Autodesk Fusion 360 part; units mm, degrees
(part 2 of 3)
component "Output_Shaft" placed x (1, 0, 0) y (0, 1, 0) z (0, 0, 1) at (0, 0, 0)
equation "d46 = d45"

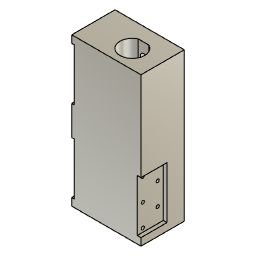
design "主轴连接"
Autodesk Fusion 360 part; units mm, degrees
sketch "草图1" plane through (0, 0, 0) normal (0, 0, 1) x (1, 0, 0)
  line L0 (4.3589, 9) -> (-4.3589, 9)
  arc A0 (-4.3589, 9) -> (4.3589, 9) centre (0, 0) ccw
  line L1 (-34, -15) -> (22, -15)
  line L2 (22, -15) -> (22, 20)
  line L3 (22, 20) -> (-34, 20)
  line L4 (-34, 20) -> (-34, -15)
  line L5 (-34, -15) -> (22, 20) construction
  line L6 (22, -15) -> (-34, 20) construction
  point P0 (-6, 2.5)
  dimension "d1" = 20
  dimension "d2" = 9
  dimension "d3" = 20
  dimension "d29" = 15
  dimension "d30" = 22
  dimension "d31" = 34
  constraint coincident A0.centre origin
  constraint horizontal L0
  constraint horizontal L1
  constraint perpendicular L1 L2
  constraint parallel L1 L3
  constraint parallel L2 L4
  constraint midpoint L5 P0
  measures "d1" diameter of A0
  measures "d2" distance of A0.centre L0
  measures "d3" distance of A0.centre L3
  measures "d29" distance of A0.centre L1
  measures "d30" distance of A0.centre L2
  measures "d31" distance of A0.centre L4
extrude "拉伸1" add sketch "草图1" along normal blind 120
sketch "草图2" plane through (0, 0, 0) normal (0, 1, 0) x (1, 0, 0)
  line L0 (0, 23.9803) -> (0, -42.7721) construction
  circle A0 centre (0, -9.3959) radius 2.5
  circle A1 centre (0, -29.3959) radius 2.5
  circle A2 centre (0, -49.3959) radius 2.5
  circle A3 centre (0, -69.3959) radius 2.5
  circle A4 centre (0, -89.3959) radius 2.5
  circle A5 centre (0, -109.3959) radius 2.5
  dimension "d7" = 5
  dimension "d10" = 20
  dimension "d11" = 0
  constraint vertical L0
  constraint coincident origin L0
  constraint midpoint L0 A0.centre
  measures "d7" diameter of A0
extrude "拉伸2" cut sketch "草图2" along normal blind 20
sketch "草图3" plane through (0, 0, 0) normal (1, 0, 0) x (0, 1, 0)
  line L0 (6, 48) -> (-15, 48)
  line L1 (-15, 48) -> (-15, 6)
  line L2 (-15, 6) -> (6, 6)
  line L3 (6, 6) -> (6, 48)
  line L4 (6, 48) -> (-15, 6) construction
  line L5 (-15, 48) -> (6, 6) construction
  line L6 (6, 114) -> (-15, 114)
  line L7 (-15, 114) -> (-15, 72)
  line L8 (-15, 72) -> (6, 72)
  line L9 (6, 72) -> (6, 114)
  line L10 (6, 114) -> (-15, 72) construction
  line L11 (-15, 114) -> (6, 72) construction
  circle A0 centre (-10.5, 27) radius 1.5
  circle A1 centre (-10.5, 9) radius 1.5
  circle A2 centre (1.5, 18) radius 1.5
  line L12 (-33.5517, 27) -> (23.4691, 27) construction
  circle A3 centre (1.5, 36) radius 1.5
  circle A4 centre (-10.5, 45) radius 1.5
  line L13 (-36.0995, 93) -> (27.7197, 93) construction
  circle A5 centre (-10.5, 93) radius 1.5
  circle A6 centre (-10.5, 75) radius 1.5
  circle A7 centre (1.5, 84) radius 1.5
  circle A8 centre (1.5, 102) radius 1.5
  circle A9 centre (-10.5, 111) radius 1.5
  point P0 (-4.5, 27)
  point P1 (-4.5, 93)
  dimension "d16" = 42
  dimension "d17" = 21
  dimension "d18" = 15
  dimension "d19" = 27
  dimension "d20" = 21
  dimension "d22" = 15
  dimension "d23" = 42
  dimension "d25" = 66
  dimension "d35" = 3
  dimension "d36" = 3
  dimension "d37" = 3
  dimension "d38" = 9
  dimension "d39" = 18
  dimension "d40" = 4.5
  dimension "d41" = 16.5
  dimension "d42" = 4.5
  dimension "d43" = 3
  dimension "d44" = 3
  dimension "d45" = 3
  dimension "d46" = 9
  dimension "d47" = 18
  dimension "d48" = 4.5
  dimension "d49" = 4.5
  dimension "d50" = 16.5
  constraint horizontal L0
  constraint perpendicular L0 L1
  constraint parallel L0 L2
  constraint parallel L1 L3
  constraint coincident L4 P0
  constraint coincident L5 P0
  constraint horizontal L6
  constraint perpendicular L6 L7
  constraint parallel L6 L8
  constraint parallel L7 L9
  constraint coincident L10 P1
  constraint coincident L11 P1
  constraint horizontal L12
  constraint coincident P0 L12
  constraint coincident A0.centre L12
  constraint symmetric A1 L12 A4
  constraint symmetric A2 L12 A3
  constraint horizontal L13
  constraint coincident P1 L13
  constraint coincident L13 A5.centre
  constraint symmetric L13 A6 A9
  constraint symmetric L13 A7 A8
  measures "d16" distance of L0.start L2.end
  measures "d17" distance of L0.start L0.end
  measures "d18" distance of origin L1
  measures "d19" vertical distance of origin P0
  measures "d20" distance of L6.start L6.end
  measures "d22" distance of origin L7
  measures "d23" distance of L6.start L8.end
  measures "d25" distance of P0 P1
  measures "d35" diameter of A0
  measures "d36" diameter of A1
  measures "d37" diameter of A2
  measures "d38" distance of A2.centre L12
  measures "d39" distance of A1.centre L12
  measures "d40" distance of L1 A0.centre
  measures "d41" distance of L1 A2.centre
  measures "d42" distance of L1 A1.centre
  measures "d43" diameter of A5
  measures "d44" diameter of A6
  measures "d45" diameter of A7
  measures "d46" distance of L13 A7.centre
  measures "d47" distance of L13 A6.centre
  measures "d48" distance of L7 A5.centre
  measures "d49" distance of L7 A6.centre
  measures "d50" distance of L7 A7.centre
extrude "拉伸3" cut sketch "草图3" along normal blind 6 from surface at 19 contours L0 L1 L2 L3 | A0 | A1 | A2 | A3 | A4
extrude "拉伸4" cut sketch "草图3" against normal blind 5 from surface at -32 contours L0 L1 L2 L3 | L6 L7 L8 L9 | A0 | A1 | A2 | A3 | A4 | A5 | A6 | A7 | A8 | A9
sketch "草图4" plane through (19, 0, 0) normal (1, 0, 0) x (0, 1, 0)
  line L0 (6, 6) -> (6, 48)
  line L1 (6, 48) -> (-15, 48)
  line L2 (-15, 48) -> (-15, 6)
  line L3 (-15, 6) -> (6, 6)
  line L4 (-15, 5.975) -> (6, 5.975)
  line L5 (-33.5517, 27) -> (23.4691, 27) construction
  line L6 (-15, 114.025) -> (6, 71.975) construction
  circle A0 centre (-10.5, 45) radius 1.5
  circle A1 centre (1.5, 102) radius 1.5
  line L7 (-15, 114.025) -> (-15, 71.975)
  line L8 (-36.0995, 93) -> (27.7197, 93) construction
  line L9 (-15, 48.025) -> (6, 5.975) construction
  line L10 (-15, 71.975) -> (6, 71.975)
  line L11 (-15, 48.025) -> (-15, 5.975)
  line L12 (6, 71.975) -> (6, 114.025)
  circle A2 centre (1.5, 84) radius 1.5
  line L13 (6, 48.025) -> (-15, 48.025)
  circle A3 centre (1.5, 18) radius 1.5
  circle A4 centre (-10.5, 9) radius 1.5
  circle A5 centre (-10.5, 93) radius 1.5
  line L14 (6, 114.025) -> (-15, 71.975) construction
  circle A6 centre (1.5, 36) radius 1.5
  line L15 (6, 114.025) -> (-15, 114.025)
  line L16 (6, 5.975) -> (6, 48.025)
  line L17 (6, 48.025) -> (-15, 5.975) construction
  circle A7 centre (-10.5, 75) radius 1.5
  circle A8 centre (-10.5, 27) radius 1.5
  circle A9 centre (-10.5, 111) radius 1.5
  point P0 (-4.5, 93)
  point P1 (-4.5, 27)
  dimension "d51" = 42.05
  dimension "d52" = 21
  dimension "d53" = 15
  dimension "d54" = 27
  dimension "d55" = 21
  dimension "d56" = 15
  dimension "d57" = 42.05
  dimension "d58" = 66
  dimension "d59" = 3
  dimension "d60" = 3
  dimension "d61" = 3
  dimension "d62" = 9
  dimension "d63" = 18
  dimension "d64" = 4.5
  dimension "d65" = 16.5
  dimension "d66" = 4.5
  dimension "d67" = 3
  dimension "d68" = 3
  dimension "d69" = 3
  dimension "d70" = 9
  dimension "d71" = 18
  dimension "d72" = 4.5
  dimension "d73" = 4.5
  dimension "d74" = 16.5
  constraint horizontal L13
  constraint perpendicular L11 L13
  constraint parallel L4 L13
  constraint parallel L11 L16
  constraint coincident P1 L17
  constraint coincident P1 L9
  constraint horizontal L15
  constraint perpendicular L7 L15
  constraint parallel L10 L15
  constraint parallel L7 L12
  constraint coincident P0 L14
  constraint coincident P0 L6
  constraint horizontal L5
  constraint coincident P1 L5
  constraint coincident A8.centre L5
  constraint symmetric L5 A0 A4
  constraint symmetric L5 A3 A6
  constraint horizontal L8
  constraint coincident P0 L8
  constraint coincident A5.centre L8
  constraint symmetric L8 A7 A9
  constraint symmetric A1 L8 A2
  measures "d51" distance of L13.start L4.end
  measures "d52" distance of L13.start L9.start
  measures "d53" distance of origin L11
  measures "d54" vertical distance of origin P1
  measures "d55" distance of L12.end L6.start
  measures "d56" distance of origin L7
  measures "d57" distance of L12.end L6.end
  measures "d58" distance of P0 P1
  measures "d59" diameter of A8
  measures "d60" diameter of A4
  measures "d61" diameter of A3
  measures "d62" distance of A3.centre L5
  measures "d63" distance of A4.centre L5
  measures "d64" distance of A8.centre L11
  measures "d65" distance of A3.centre L11
  measures "d66" distance of A4.centre L11
  measures "d67" diameter of A5
  measures "d68" diameter of A7
  measures "d69" diameter of A2
  measures "d70" distance of A2.centre L8
  measures "d71" distance of A7.centre L8
  measures "d72" distance of A5.centre L7
  measures "d73" distance of A7.centre L7
  measures "d74" distance of A2.centre L7
sketch "草图5" plane through (-32, 0, 0) normal (-1, 0, 0) x (0, -1, 0)
  line L0 (-6, 48) -> (-6, 6)
  line L1 (-6, 6) -> (15, 6)
  line L2 (15, 6) -> (15, 48)
  line L3 (15, 48) -> (-6, 48)
  line L4 (15, 5.975) -> (-6, 5.975)
  line L5 (33.5517, 27) -> (-23.4691, 27) construction
  line L6 (15, 114.025) -> (-6, 71.975) construction
  circle A0 centre (10.5, 45) radius 1.5
  circle A1 centre (-1.5, 102) radius 1.5
  line L7 (15, 114.025) -> (15, 71.975)
  line L8 (36.0995, 93) -> (-27.7197, 93) construction
  line L9 (15, 48.025) -> (-6, 5.975) construction
  line L10 (15, 71.975) -> (-6, 71.975)
  line L11 (15, 48.025) -> (15, 5.975)
  line L12 (-6, 71.975) -> (-6, 114.025)
  circle A2 centre (-1.5, 84) radius 1.5
  line L13 (-6, 48.025) -> (15, 48.025)
  circle A3 centre (-1.5, 18) radius 1.5
  circle A4 centre (10.5, 9) radius 1.5
  circle A5 centre (10.5, 93) radius 1.5
  line L14 (-6, 114.025) -> (15, 71.975) construction
  circle A6 centre (-1.5, 36) radius 1.5
  line L15 (-6, 114.025) -> (15, 114.025)
  line L16 (-6, 5.975) -> (-6, 48.025)
  line L17 (-6, 48.025) -> (15, 5.975) construction
  circle A7 centre (10.5, 75) radius 1.5
  circle A8 centre (10.5, 27) radius 1.5
  circle A9 centre (10.5, 111) radius 1.5
  point P0 (4.5, 93)
  point P1 (4.5, 27)
  dimension "d75" = 42.05
  dimension "d76" = 21
  dimension "d77" = 15
  dimension "d79" = 21
  dimension "d80" = 15
  dimension "d81" = 42.05
  dimension "d82" = 66
  dimension "d83" = 3
  dimension "d84" = 3
  dimension "d85" = 3
  dimension "d86" = 9
  dimension "d87" = 18
  dimension "d88" = 4.5
  dimension "d89" = 16.5
  dimension "d90" = 4.5
  dimension "d91" = 3
  dimension "d92" = 3
  dimension "d93" = 3
  dimension "d94" = 9
  dimension "d95" = 18
  dimension "d96" = 4.5
  dimension "d97" = 4.5
  dimension "d98" = 16.5
  constraint perpendicular L11 L13
  constraint parallel L4 L13
  constraint parallel L11 L16
  constraint coincident P1 L17
  constraint coincident P1 L9
  constraint perpendicular L7 L15
  constraint parallel L10 L15
  constraint parallel L7 L12
  constraint coincident P0 L14
  constraint coincident P0 L6
  constraint coincident P1 L5
  constraint coincident A8.centre L5
  constraint symmetric L5 A0 A4
  constraint symmetric L5 A3 A6
  constraint coincident P0 L8
  constraint coincident A5.centre L8
  constraint symmetric L8 A7 A9
  constraint symmetric A1 L8 A2
  measures "d75" distance of L13.start L4.end
  measures "d76" distance of L13.start L9.start
  measures "d77" distance of origin L11
  measures "d79" distance of L12.end L6.start
  measures "d80" distance of origin L7
  measures "d81" distance of L12.end L6.end
  measures "d82" distance of P0 P1
  measures "d83" diameter of A8
  measures "d84" diameter of A4
  measures "d85" diameter of A3
  measures "d86" distance of A3.centre L5
  measures "d87" distance of A4.centre L5
  measures "d88" distance of A8.centre L11
  measures "d89" distance of A3.centre L11
  measures "d90" distance of A4.centre L11
  measures "d91" diameter of A5
  measures "d92" diameter of A7
  measures "d93" diameter of A2
  measures "d94" distance of A2.centre L8
  measures "d95" distance of A7.centre L8
  measures "d96" distance of A5.centre L7
  measures "d97" distance of A7.centre L7
  measures "d98" distance of A2.centre L7
hole "孔1" at (19, 1.5, 18) at (19, -10.5, 9) at (19, -10.5, 27) at (19, 1.5, 36) at (19, -10.5, 45) direction (-1, 0, 0) diameter 2.529 depth 6 tip angle 180
thread "螺纹1" "ISO Metric profile 3.0 M3x0.5 6H" major diameter 3.086 minor diameter 2.529 pitch 0.5 angle 60 resizes the face on face at (15, 1.6259, 16.7418) on face at (15, -10.3741, 25.7418) on face at (17, 0.2359, 36.0315) on face at (15, -10.3741, 7.7418) on face at (17, -11.7641, 45.0315)
hole "孔2" at (-32, -10.5, 9) at (-32, -10.5, 27) at (-32, 1.5, 18) at (-32, 1.5, 36) at (-32, -10.5, 45) at (-32, -10.5, 75) at (-32, 1.5, 84) at (-32, -10.5, 93) at (-32, 1.5, 102) at (-32, -10.5, 111) direction (1, 0, 0) diameter 2.529 depth 6 tip angle 180
thread "螺纹2" "ISO Metric profile 3.0 M3x0.5 6H" major diameter 3.086 minor diameter 2.529 pitch 0.5 angle 60 resizes the face on face at (-30, -11.7547, 111.1572) on face at (-30, -11.7547, 93.1572) on face at (-30, -11.7547, 75.1572) on face at (-28, -10.3741, 28.2582) on face at (-28, -10.3741, 10.2582) on face at (-28, 1.6259, 19.2582) on face at (-30, 0.2453, 84.1572) on face at (-30, 0.2359, 35.9685) on face at (-30, -11.7641, 44.9685) on face at (-30, 0.2453, 102.1572)

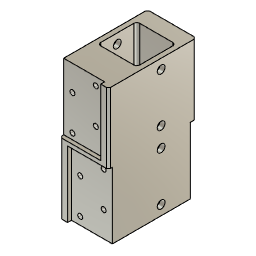
design "铝型连42"
Autodesk Fusion 360 part; units mm, degrees
sketch "草图1" plane through (0, 0, 0) normal (0, 0, 1) x (1, 0, 0)
  line L0 (8.5, 10) -> (-8.5, 10)
  line L1 (-10, 8.5) -> (-10, -8.5)
  line L2 (-8.5, -10) -> (8.5, -10)
  line L3 (10, -8.5) -> (10, 8.5)
  line L4 (10, 10) -> (-10, -10) construction
  line L5 (-10, 10) -> (10, -10) construction
  line L6 (11.5, 18) -> (-11.5, 18)
  line L7 (-12.5, 17) -> (-12.5, -26)
  line L8 (-11.5, -27) -> (11.5, -27)
  line L9 (12.5, -26) -> (12.5, 17)
  line L10 (12.5, 18) -> (-12.5, -27) construction
  line L11 (-12.5, 18) -> (12.5, -27) construction
  arc A0 (10, 8.5) -> (8.5, 10) centre (8.5, 8.5) ccw
  arc A1 (8.5, -10) -> (10, -8.5) centre (8.5, -8.5) ccw
  arc A2 (-10, -8.5) -> (-8.5, -10) centre (-8.5, -8.5) ccw
  arc A3 (-8.5, 10) -> (-10, 8.5) centre (-8.5, 8.5) ccw
  line L12 (11.5, 18) -> (12.5, 17)
  line L13 (12.5, -26) -> (11.5, -27)
  line L14 (-11.5, -27) -> (-12.5, -26)
  line L15 (-12.5, 17) -> (-11.5, 18)
  line L16 (0, -4.5) -> (0, 0) construction
  point P0 (0, -4.5)
  dimension "d2" = 20
  dimension "d3" = 25
  dimension "d4" = 1.5
  dimension "d5" = 1
  dimension "d6" = 1
  dimension "d7" = 1
  dimension "d8" = 1
  dimension "d9" = 1
  dimension "d10" = 1
  dimension "d11" = 1
  dimension "d12" = 1
  dimension "d138" = 20
  dimension "d139" = 20
  dimension "d140" = 45
  dimension "d141" = 18
  constraint horizontal L0
  constraint perpendicular L0 L1
  constraint parallel L0 L2
  constraint parallel L1 L3
  constraint coincident L4 L16.end
  constraint coincident L5 L16.end
  constraint coincident L16.end origin
  constraint horizontal L6
  constraint perpendicular L6 L7
  constraint parallel L6 L8
  constraint parallel L7 L9
  constraint coincident L4.start L0
  constraint coincident L4.start L3
  constraint tangent L0 A0
  constraint tangent L3 A0
  constraint coincident L5.end L3
  constraint coincident L5.end L2
  constraint tangent L3 A1
  constraint tangent L2 A1
  constraint equal A0 A1
  constraint coincident L4.end L2
  constraint coincident L4.end L1
  constraint tangent L2 A2
  constraint tangent L1 A2
  constraint equal A0 A2
  constraint coincident L5.start L1
  constraint coincident L5.start L0
  constraint tangent L1 A3
  constraint tangent L0 A3
  constraint equal A0 A3
  constraint coincident L10.start L6
  constraint coincident L10.start L9
  constraint coincident L11.end L9
  constraint coincident L11.end L8
  constraint coincident L10.end L8
  constraint coincident L10.end L7
  constraint coincident L11.start L7
  constraint coincident L11.start L6
  constraint midpoint L11 P0
  constraint coincident P0 L16.start
  constraint vertical L16
  measures "d2" distance of L4.start L5.start
  measures "d3" distance of L10.start L11.start
  measures "d4" radius of A0
  measures "d5" distance of L10.start L6.start
  measures "d6" distance of L10.start L9.end
  measures "d7" distance of L11.end L9.start
  measures "d8" distance of L11.end L8.end
  measures "d9" distance of L10.end L8.start
  measures "d10" distance of L10.end L7.end
  measures "d11" distance of L11.start L7.start
  measures "d12" distance of L11.start L6.end
  measures "d138" distance of L0 L2
  measures "d139" distance of L1 L3
  measures "d140" distance of L6 L8
  measures "d141" distance of L16.end L6
extrude "拉伸1" add sketch "草图1" along normal blind 70
sketch "草图17" plane through (0, 0, 0) normal (1, 0, 0) x (0, 1, 0)
  line L0 (0, 80.0802) -> (0, -28.3534) construction
  circle A0 centre (0, 5) radius 2
  circle A1 centre (0, 30) radius 2
  circle A2 centre (0, 40) radius 2
  circle A3 centre (0, 65) radius 2
  line L1 (17, 70) -> (-26, 70)
  dimension "d229" = 4
  dimension "d230" = 4
  dimension "d231" = 5
  dimension "d232" = 30
  dimension "d239" = 4
  dimension "d240" = 4
  dimension "d241" = 5
  dimension "d242" = 30
  constraint vertical L0
  constraint coincident L0 origin
  constraint coincident L0 A0.centre
  constraint coincident L0 A1.centre
  constraint coincident L0 A2.centre
  constraint coincident L0 A3.centre
  measures "d229" diameter of A1
  measures "d230" diameter of A0
  measures "d231" distance of origin A0.centre
  measures "d232" distance of origin A1.centre
  measures "d239" diameter of A2
  measures "d240" diameter of A3
  measures "d241" distance of A3.centre L1
  measures "d242" distance of A2.centre L1
extrude "拉伸16" cut sketch "草图17" along normal mid plane 40
sketch "草图2" plane through (0, 0, 0) normal (0, 1, 0) x (1, 0, 0)
  line L0 (-20, -13) -> (68.6106, -13)
  line L1 (33.5, -65) -> (33.5, 25)
  line L2 (-72.1271, -53) -> (20, -53)
  line L3 (-33.5, -85) -> (-33.5, -15)
  point P0 (33.5, -13)
  point P1 (-33.5, -53)
  dimension "d15" = 33.5
  dimension "d16" = 33.5
  dimension "d17" = 13
  dimension "d18" = 53
  dimension "d19" = 78.032
  constraint horizontal L0
  constraint vertical L1
  constraint horizontal L2
  constraint vertical L3
  constraint coincident L1 P0
  constraint coincident L0 P0
  constraint coincident L2 P1
  constraint coincident L3 P1
  measures "d15" distance of origin L1
  measures "d16" distance of origin L3
  measures "d17" distance of origin L0
  measures "d18" distance of origin L2
  measures "d19" distance of P0 P1
sketch "草图14" plane through (0, 0, 0) normal (0, 1, 0) x (1, 0, 0)
  line L0 (-8.5, -34) -> (12.5, -34)
  line L1 (12.5, -34) -> (12.5, 8)
  line L2 (12.5, 8) -> (-8.5, 8)
  line L3 (-8.5, 8) -> (-8.5, -34)
  line L4 (-8.5, -34) -> (12.5, 8) construction
  line L5 (12.5, -34) -> (-8.5, 8) construction
  line L6 (-12.5, -78) -> (8.5, -78)
  line L7 (8.5, -78) -> (8.5, -36)
  line L8 (8.5, -36) -> (-12.5, -36)
  line L9 (-12.5, -36) -> (-12.5, -78)
  line L10 (-12.5, -78) -> (8.5, -36) construction
  line L11 (8.5, -78) -> (-12.5, -36) construction
  circle A0 centre (8, 5) radius 1.5
  line L12 (21.5, -13) -> (-20.5, -13) construction
  circle A1 centre (8, -13) radius 1.5
  circle A2 centre (-4, -4) radius 1.5
  circle A3 centre (-4, -22) radius 1.5
  circle A4 centre (8, -31) radius 1.5
  line L13 (17.5, -57) -> (-26.5, -57) construction
  circle A5 centre (-8, -39) radius 1.5
  circle A6 centre (4, -48) radius 1.5
  circle A7 centre (-8, -57) radius 1.5
  circle A8 centre (-8, -75) radius 1.5
  circle A9 centre (4, -66) radius 1.5
  point P0 (2, -13)
  point P1 (-2, -57)
  dimension "d145" = 21
  dimension "d146" = 42
  dimension "d147" = 12.5
  dimension "d148" = 42
  dimension "d149" = 21
  dimension "d150" = 12.5
  dimension "d151" = 13
  dimension "d152" = 57
  dimension "d153" = 3
  dimension "d154" = 3
  dimension "d155" = 3
  dimension "d156" = 4.5
  dimension "d157" = 4.5
  dimension "d158" = 16.5
  dimension "d159" = 9
  dimension "d160" = 18
  dimension "d161" = 3
  dimension "d162" = 3
  dimension "d163" = 3
  dimension "d164" = 18
  dimension "d165" = 9
  dimension "d166" = 4.5
  dimension "d167" = 16.5
  dimension "d168" = 4.5
  constraint horizontal L0
  constraint perpendicular L0 L1
  constraint parallel L0 L2
  constraint parallel L1 L3
  constraint coincident L4 P0
  constraint coincident L5 P0
  constraint horizontal L6
  constraint perpendicular L6 L7
  constraint parallel L6 L8
  constraint parallel L7 L9
  constraint coincident L10 P1
  constraint coincident L11 P1
  constraint perpendicular L1 L12
  constraint coincident P0 L12
  constraint coincident L12 A1.centre
  constraint symmetric A0 L12 A4
  constraint symmetric L12 A2 A3
  constraint horizontal L13
  constraint coincident P1 L13
  constraint coincident L13 A7.centre
  constraint symmetric L13 A5 A8
  constraint symmetric L13 A6 A9
  measures "d145" distance of L1.end L2.end
  measures "d146" distance of L0.end L1.end
  measures "d147" distance of origin L1
  measures "d148" distance of L6.start L8.end
  measures "d149" distance of L6.start L6.end
  measures "d150" distance of origin L9
  measures "d151" vertical distance of origin P0
  measures "d152" vertical distance of origin P1
  measures "d153" diameter of A0
  measures "d154" diameter of A2
  measures "d155" diameter of A1
  measures "d156" distance of L1 A0.centre
  measures "d157" distance of L1 A1.centre
  measures "d158" distance of L1 A2.centre
  measures "d159" distance of L12 A2.centre
  measures "d160" distance of A0.centre L12
  measures "d161" diameter of A7
  measures "d162" diameter of A5
  measures "d163" diameter of A6
  measures "d164" distance of L13 A5.centre
  measures "d165" distance of L13 A6.centre
  measures "d166" distance of L9 A7.centre
  measures "d167" distance of L9 A6.centre
  measures "d168" distance of L9 A5.centre
extrude "拉伸14" cut sketch "草图14" against normal blind 3 from surface at 18 contours L0 L1 L2 L3 | A0 | A1 | A2 | A3 | A4
extrude "拉伸15" cut sketch "草图14" along normal blind 2 from surface at -27 contours L0 L1 L2 L3 | L6 L7 L8 L9 | A0 | A1 | A2 | A3 | A4 | A5 | A6 | A7 | A8 | A9
sketch "草图15" plane through (0, 15, 0) normal (0, 1, 0) x (-1, 0, 0)
  line L0 (-12.5, 0) -> (8.5, 0)
  line L1 (8.5, 0) -> (8.5, 34)
  line L2 (8.5, 34) -> (-12.5, 34)
  line L3 (-8.5, 36) -> (12.5, 36)
  circle A0 centre (-8, 13) radius 1.5
  line L4 (8.5, 34) -> (-12.5, 34)
  line L5 (-8.5, 36) -> (12.5, 78) construction
  line L6 (12.5, 36) -> (-8.5, 78) construction
  line L7 (17, 13) -> (-27, 13) construction
  circle A1 centre (8, 39) radius 1.5
  line L8 (-8.5, 78) -> (-8.5, 36)
  circle A2 centre (4, 22) radius 1.5
  line L9 (12.5, 78) -> (-8.5, 78)
  line L10 (8.5, -8) -> (8.5, 34)
  line L11 (-12.5, -8) -> (8.5, 34) construction
  line L12 (12.5, 36) -> (12.5, 78)
  circle A3 centre (-4, 66) radius 1.5
  circle A4 centre (8, 57) radius 1.5
  circle A5 centre (8, 75) radius 1.5
  circle A6 centre (-8, -5) radius 1.5
  line L13 (-12.5, 34) -> (-12.5, -8)
  line L14 (8.5, -8) -> (-12.5, 34) construction
  line L15 (-12.5, -8) -> (8.5, -8)
  circle A7 centre (-4, 48) radius 1.5
  line L16 (21, 57) -> (-21, 57) construction
  circle A8 centre (4, 4) radius 1.5
  circle A9 centre (-8, 31) radius 1.5
  line L17 (-12.5, 34) -> (-12.5, 0)
  point P0 (2, 57)
  point P1 (0, 70)
  point P2 (-2, 13)
  dimension "d172" = 21
  dimension "d173" = 42
  dimension "d174" = 12.5
  dimension "d175" = 42
  dimension "d176" = 21
  dimension "d177" = 12.5
  dimension "d178" = 13
  dimension "d180" = 3
  dimension "d181" = 3
  dimension "d182" = 3
  dimension "d183" = 4.5
  dimension "d184" = 4.5
  dimension "d185" = 16.5
  dimension "d186" = 9
  dimension "d187" = 18
  dimension "d188" = 3
  dimension "d189" = 3
  dimension "d190" = 3
  dimension "d191" = 18
  dimension "d192" = 9
  dimension "d193" = 4.5
  dimension "d194" = 16.5
  dimension "d195" = 4.5
  dimension "d235" = 57
  dimension "d238" = 13
  constraint horizontal L3
  constraint perpendicular L3 L12
  constraint parallel L3 L9
  constraint parallel L8 L12
  constraint coincident P0 L5
  constraint coincident P0 L6
  constraint horizontal L15
  constraint perpendicular L10 L15
  constraint parallel L4 L15
  constraint parallel L10 L13
  constraint coincident P2 L11
  constraint coincident P2 L14
  constraint perpendicular L12 L16
  constraint coincident P0 L16
  constraint coincident A4.centre L16
  constraint symmetric A1 A5 L16
  constraint symmetric A3 A7 L16
  constraint horizontal L7
  constraint coincident P2 L7
  constraint coincident A0.centre L7
  constraint symmetric L7 A6 A9
  constraint symmetric L7 A2 A8
  measures "d172" distance of L5.end L6.end
  measures "d173" distance of L5.end L3.end
  measures "d174" distance of origin L12
  measures "d175" distance of L11.start L2.end
  measures "d176" distance of L11.start L10.start
  measures "d177" distance of origin L13
  measures "d178" vertical distance of P0 P1
  measures "d180" diameter of A5
  measures "d181" diameter of A3
  measures "d182" diameter of A4
  measures "d183" distance of A5.centre L12
  measures "d184" distance of A4.centre L12
  measures "d185" distance of A3.centre L12
  measures "d186" distance of A3.centre L16
  measures "d187" distance of A5.centre L16
  measures "d188" diameter of A0
  measures "d189" diameter of A9
  measures "d190" diameter of A2
  measures "d191" distance of A9.centre L7
  measures "d192" distance of A2.centre L7
  measures "d193" distance of A0.centre L13
  measures "d194" distance of A2.centre L13
  measures "d195" distance of A9.centre L13
  measures "d235" vertical distance of origin P0
  measures "d238" vertical distance of origin P2
hole "孔2" at (-4, 15, 22) at (8, 15, 31) at (8, 15, 13) at (-4, 15, 4) at (8, 15, -5) direction (0, -1, 0) diameter 2.529 depth 5 tip angle 118
thread "螺纹1" "ISO Metric profile 3.0 M3x0.5 6H" major diameter 3.086 minor diameter 2.529 pitch 0.5 angle 60 resizes the face on face at (-3.937, 13.3333, 5.2629) on face at (-3.937, 13.3333, 23.2629) on face at (9.2645, 13.3333, 13) on face at (9.2645, 13.3333, 31)
sketch "草图16" plane through (0, -25, 0) normal (0, -1, 0) x (1, 0, 0)
  line L0 (8.5, 70) -> (-12.5, 70)
  line L1 (-12.5, 36) -> (8.5, 36)
  line L2 (-8.5, 34) -> (-8.5, 0)
  line L3 (-8.5, 0) -> (12.5, 0)
  line L4 (12.5, 34) -> (-8.5, 34)
  line L5 (8.5, 36) -> (8.5, 70)
  line L6 (12.5, -8) -> (-8.5, -8)
  line L7 (-12.5, 78) -> (8.5, 78)
  line L8 (-8.5, -8) -> (12.5, 34) construction
  circle A0 centre (8, 13) radius 1.5
  circle A1 centre (-8, 39) radius 1.5
  circle A2 centre (4, 66) radius 1.5
  line L9 (-12.5, 36) -> (-12.5, 78)
  line L10 (12.5, 34) -> (12.5, -8)
  circle A3 centre (-8, 75) radius 1.5
  circle A4 centre (-4, 4) radius 1.5
  line L11 (-25.9432, 13) -> (38.5312, 13) construction
  line L12 (-12.5, 36) -> (8.5, 78) construction
  line L13 (8.5, 36) -> (-12.5, 78) construction
  circle A5 centre (8, 31) radius 1.5
  line L14 (8.5, 78) -> (8.5, 36)
  circle A6 centre (8, -5) radius 1.5
  line L15 (-52.1531, 57) -> (39, 57) construction
  line L16 (8.5, 36) -> (-12.5, 36)
  line L17 (-8.5, -8) -> (-8.5, 34)
  circle A7 centre (-8, 57) radius 1.5
  line L18 (12.5, -8) -> (-8.5, 34) construction
  line L19 (-8.5, 34) -> (12.5, 34)
  circle A8 centre (-4, 22) radius 1.5
  circle A9 centre (4, 48) radius 1.5
  line L20 (12.5, 0) -> (12.5, 34)
  line L21 (-12.5, 70) -> (-12.5, 36)
  point P0 (-2, 57)
  point P1 (0, 68)
  point P2 (2, 13)
  dimension "d202" = 21
  dimension "d203" = 42
  dimension "d204" = 12.5
  dimension "d205" = 42
  dimension "d206" = 21
  dimension "d207" = 12.5
  dimension "d210" = 3
  dimension "d211" = 3
  dimension "d212" = 3
  dimension "d213" = 4.5
  dimension "d214" = 4.5
  dimension "d215" = 16.5
  dimension "d216" = 9
  dimension "d217" = 18
  dimension "d218" = 3
  dimension "d219" = 3
  dimension "d220" = 3
  dimension "d221" = 18
  dimension "d222" = 9
  dimension "d223" = 4.5
  dimension "d224" = 16.5
  dimension "d225" = 4.5
  dimension "d236" = 13
  dimension "d237" = 57
  constraint perpendicular L9 L16
  constraint parallel L7 L16
  constraint parallel L9 L14
  constraint coincident P0 L13
  constraint coincident P0 L12
  constraint perpendicular L6 L17
  constraint parallel L6 L19
  constraint parallel L10 L17
  constraint coincident P2 L18
  constraint coincident P2 L8
  constraint perpendicular L9 L15
  constraint coincident P0 L15
  constraint coincident A7.centre L15
  constraint symmetric A1 A3 L15
  constraint symmetric A2 L15 A9
  constraint coincident P2 L11
  constraint coincident A0.centre L11
  constraint symmetric L11 A5 A6
  constraint symmetric A4 L11 A8
  constraint horizontal L7
  constraint horizontal L19
  constraint horizontal L11
  measures "d202" distance of L7.start L7.end
  measures "d203" distance of L7.start L1.start
  measures "d204" distance of origin L9
  measures "d205" distance of L6.start L4.start
  measures "d206" distance of L6.start L6.end
  measures "d207" distance of origin L10
  measures "d210" diameter of A3
  measures "d211" diameter of A2
  measures "d212" diameter of A7
  measures "d213" distance of A3.centre L9
  measures "d214" distance of A7.centre L9
  measures "d215" distance of A2.centre L9
  measures "d216" distance of A2.centre L15
  measures "d217" distance of A3.centre L15
  measures "d218" diameter of A0
  measures "d219" diameter of A5
  measures "d220" diameter of A8
  measures "d221" distance of A5.centre L11
  measures "d222" distance of A8.centre L11
  measures "d223" distance of A0.centre L10
  measures "d224" distance of A8.centre L10
  measures "d225" distance of A5.centre L10
  measures "d236" distance of origin L11
  measures "d237" distance of origin L15
hole "孔3" at (4, -25, 66) at (-8, -25, 57) at (4, -25, 48) at (-8, -25, 39) at (8, -25, 31) at (-4, -25, 22) at (8, -25, 13) at (-4, -25, 4) direction (0, 1, 0) diameter 2.529 depth 6 tip angle 118
thread "螺纹2" "ISO Metric profile 3.0 M3x0.5 6H" major diameter 3.086 minor diameter 2.529 pitch 0.5 angle 60 resizes the face on face at (8.1259, -21, 11.7418) on face at (2.7453, -23, 65.8428) on face at (-3.8741, -21, 2.7418) on face at (-9.2641, -23, 39.0315) on face at (2.7359, -23, 48.0315) on face at (-9.2641, -23, 57.0315) on face at (8.1259, -21, 29.7418) on face at (-3.8741, -21, 20.7418)
equation "d6 = d5"
equation "d8 = d7"
equation "d10 = d9"
equation "d12 = d11"

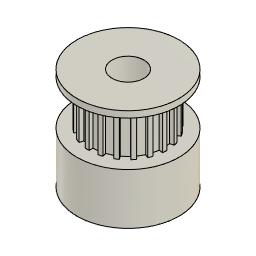
design "2GT20同步轮"
Autodesk Fusion 360 part; units mm, degrees
sketch "草图1" plane through (0, 0, 0) normal (0, 0, 1) x (1, 0, 0)
  circle A0 centre (0, 0) radius 8
  circle A1 centre (0, 0) radius 2.5
  dimension "d1" = 16
  dimension "d2" = 5
  constraint coincident A0.centre A1.centre
  measures "d1" diameter of A0
  measures "d2" diameter of A1
extrude "拉伸1" add sketch "草图1" along normal blind 16
sketch "草图2" plane through (0, 0, 0) normal (0, 0, 1) x (1, 0, 0)
  circle A0 centre (0, 0) radius 8
  line L0 (0, 0) -> (1.8881, 5.811) construction
  line L1 (0, 0) -> (0, 6.11) construction
  line L2 (1.8889, 5.8134) -> (1.6996, 5.2308)
  line L3 (1.6996, 5.2308) -> (0.5749, 5.4699)
  line L4 (0.6387, 6.0765) -> (0, 6.1126)
  line L5 (0.6387, 6.0765) -> (0, 0) construction
  line L6 (0.6387, 6.0765) -> (0.5749, 5.4699)
  line L7 (0.6387, 6.0765) -> (0.5749, 5.4699)
  line L8 (-1.2703, 5.9765) -> (-1.8889, 5.8134)
  line L9 (-1.2703, 5.9765) -> (-1.1435, 5.3798)
  line L10 (0, 5.5) -> (-1.1435, 5.3798)
  line L11 (0, 6.1126) -> (0, 5.5)
  line L12 (-3.055, 5.2914) -> (-3.5929, 4.9452)
  line L13 (-3.055, 5.2914) -> (-2.75, 4.7631)
  line L14 (-1.6996, 5.2308) -> (-2.75, 4.7631)
  line L15 (-1.8889, 5.8134) -> (-1.6996, 5.2308)
  line L16 (-4.5406, 4.0884) -> (-4.9452, 3.5929)
  line L17 (-4.5406, 4.0884) -> (-4.0873, 3.6802)
  line L18 (-3.2328, 4.4496) -> (-4.0873, 3.6802)
  line L19 (-3.5929, 4.9452) -> (-3.2328, 4.4496)
  line L20 (-5.5818, 2.4852) -> (-5.8134, 1.8889)
  line L21 (-5.5818, 2.4852) -> (-5.0245, 2.2371)
  line L22 (-4.4496, 3.2328) -> (-5.0245, 2.2371)
  line L23 (-4.9452, 3.5929) -> (-4.4496, 3.2328)
  line L24 (-6.0765, 0.6387) -> (-6.1126, 0)
  line L25 (-6.0765, 0.6387) -> (-5.4699, 0.5749)
  line L26 (-5.2308, 1.6996) -> (-5.4699, 0.5749)
  line L27 (-5.8134, 1.8889) -> (-5.2308, 1.6996)
  line L28 (-5.9765, -1.2703) -> (-5.8134, -1.8889)
  line L29 (-5.9765, -1.2703) -> (-5.3798, -1.1435)
  line L30 (-5.5, 0) -> (-5.3798, -1.1435)
  line L31 (-6.1126, 0) -> (-5.5, 0)
  line L32 (-5.2914, -3.055) -> (-4.9452, -3.5929)
  line L33 (-5.2914, -3.055) -> (-4.7631, -2.75)
  line L34 (-5.2308, -1.6996) -> (-4.7631, -2.75)
  line L35 (-5.8134, -1.8889) -> (-5.2308, -1.6996)
  line L36 (-4.0884, -4.5406) -> (-3.5929, -4.9452)
  line L37 (-4.0884, -4.5406) -> (-3.6802, -4.0873)
  line L38 (-4.4496, -3.2328) -> (-3.6802, -4.0873)
  line L39 (-4.9452, -3.5929) -> (-4.4496, -3.2328)
  line L40 (-2.4852, -5.5818) -> (-1.8889, -5.8134)
  line L41 (-2.4852, -5.5818) -> (-2.2371, -5.0245)
  line L42 (-3.2328, -4.4496) -> (-2.2371, -5.0245)
  line L43 (-3.5929, -4.9452) -> (-3.2328, -4.4496)
  line L44 (-0.6387, -6.0765) -> (0, -6.1126)
  line L45 (-0.6387, -6.0765) -> (-0.5749, -5.4699)
  line L46 (-1.6996, -5.2308) -> (-0.5749, -5.4699)
  line L47 (-1.8889, -5.8134) -> (-1.6996, -5.2308)
  line L48 (1.2703, -5.9765) -> (1.8889, -5.8134)
  line L49 (1.2703, -5.9765) -> (1.1435, -5.3798)
  line L50 (0, -5.5) -> (1.1435, -5.3798)
  line L51 (0, -6.1126) -> (0, -5.5)
  line L52 (3.055, -5.2914) -> (3.5929, -4.9452)
  line L53 (3.055, -5.2914) -> (2.75, -4.7631)
  line L54 (1.6996, -5.2308) -> (2.75, -4.7631)
  line L55 (1.8889, -5.8134) -> (1.6996, -5.2308)
  line L56 (4.5406, -4.0884) -> (4.9452, -3.5929)
  line L57 (4.5406, -4.0884) -> (4.0873, -3.6802)
  line L58 (3.2328, -4.4496) -> (4.0873, -3.6802)
  line L59 (3.5929, -4.9452) -> (3.2328, -4.4496)
  line L60 (5.5818, -2.4852) -> (5.8134, -1.8889)
  line L61 (5.5818, -2.4852) -> (5.0245, -2.2371)
  line L62 (4.4496, -3.2328) -> (5.0245, -2.2371)
  line L63 (4.9452, -3.5929) -> (4.4496, -3.2328)
  line L64 (6.0765, -0.6387) -> (6.1126, 0)
  line L65 (6.0765, -0.6387) -> (5.4699, -0.5749)
  line L66 (5.2308, -1.6996) -> (5.4699, -0.5749)
  line L67 (5.8134, -1.8889) -> (5.2308, -1.6996)
  line L68 (5.9765, 1.2703) -> (5.8134, 1.8889)
  line L69 (5.9765, 1.2703) -> (5.3798, 1.1435)
  line L70 (5.5, 0) -> (5.3798, 1.1435)
  line L71 (6.1126, 0) -> (5.5, 0)
  line L72 (5.2914, 3.055) -> (4.9452, 3.5929)
  line L73 (5.2914, 3.055) -> (4.7631, 2.75)
  line L74 (5.2308, 1.6996) -> (4.7631, 2.75)
  line L75 (5.8134, 1.8889) -> (5.2308, 1.6996)
  line L76 (4.0884, 4.5406) -> (3.5929, 4.9452)
  line L77 (4.0884, 4.5406) -> (3.6802, 4.0873)
  line L78 (4.4496, 3.2328) -> (3.6802, 4.0873)
  line L79 (4.9452, 3.5929) -> (4.4496, 3.2328)
  line L80 (2.4852, 5.5818) -> (1.8889, 5.8134)
  line L81 (2.4852, 5.5818) -> (2.2371, 5.0245)
  line L82 (3.2328, 4.4496) -> (2.2371, 5.0245)
  line L83 (3.5929, 4.9452) -> (3.2328, 4.4496)
  dimension "d5" = 16
  dimension "d6" = 18
  dimension "d7" = 6.11
  dimension "d12" = 360
  dimension "d16" = 5.5
  dimension "d17" = 5.5
  dimension "d19" = 6
  constraint coincident A0.centre L0.start
  constraint vertical L1
  constraint coincident L0 L2.end
  constraint parallel L0 L2
  constraint coincident L5 L3.end
  constraint equal L1 L5
  constraint equal L0 L1
  measures "d5" diameter of A0
  measures "d6" angle of L0 L1
  measures "d7" distance of A0.centre L1.end
  measures "d16" distance of A0.centre L3.end
  measures "d17" distance of A0.centre L2.end
  measures "d19" angle of L1 L6
extrude "拉伸2" cut sketch "草图2" along normal blind 7 from surface at 8

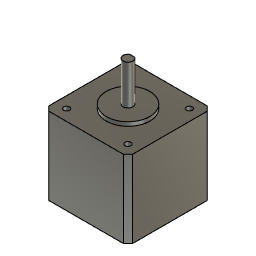
design "42*39stepper"
Autodesk Fusion 360 part; units mm, degrees
sketch "Sketch1" plane through (0, 0, 0) normal (0, 0, 1) x (1, 0, 0)
  line L0 (18.85, -21.15) -> (-18.85, -21.15)
  line L1 (-21.15, -18.85) -> (-21.15, 18.85)
  line L2 (-18.85, 21.15) -> (18.85, 21.15)
  line L3 (21.15, 18.85) -> (21.15, -18.85)
  line L4 (21.15, -21.15) -> (-21.15, 21.15) construction
  line L5 (-21.15, -21.15) -> (21.15, 21.15) construction
  line L6 (-21.15, 18.85) -> (-18.85, 21.15)
  line L7 (21.15, 21.15) -> (21.15, 18.85)
  line L8 (18.85, 21.15) -> (21.15, 18.85)
  line L9 (18.85, -21.15) -> (21.15, -18.85)
  line L10 (-21.15, -18.85) -> (-18.85, -21.15)
  line L11 (-14, 15.5) -> (-15.5, 15.5)
  circle A0 centre (-15.5, 15.5) radius 1.5
  circle A1 centre (15.5, 15.5) radius 1.5
  circle A2 centre (-15.5, -15.5) radius 1.5
  circle A3 centre (15.5, -15.5) radius 1.5
  dimension "d1" = 42.3
  dimension "d2" = 42.3
  dimension "d3" = 2.3
  dimension "d4" = 2.3
  dimension "d5" = 2.3
  dimension "d6" = 2.3
  dimension "d9" = 3
  dimension "d10" = 21.9203
  dimension "d13" = 31
  dimension "d14" = -31
  constraint horizontal L0
  constraint perpendicular L0 L1
  constraint parallel L0 L2
  constraint parallel L1 L3
  constraint coincident L4 origin
  constraint coincident L5 origin
  constraint symmetric L5 L2.start L3.end
  constraint symmetric L5 L1.end L0.start
  constraint symmetric L4 L2.end L1.start
  constraint symmetric L4 L3.start L0.end
  constraint coincident L11.end A0.centre
  constraint coincident A0 L11.start
  measures "d1" distance of L4.end L5.end
  measures "d2" distance of L5.start L4.end
  measures "d3" distance of L4.end L2.start
  measures "d4" distance of L4.end L1.end
  measures "d5" distance of L5.end L2.end
  measures "d6" distance of L5.end L3.start
  measures "d9" diameter of A0
  measures "d10" distance of origin L11.end
extrude "Extrude1" add sketch "Sketch1" along normal mid plane 39
sketch "Sketch2" plane through (0, 0, 19.5) normal (0, 0, 1) x (-1, 0, 0)
  circle A0 centre (15.5, -15.5) radius 1.5
  circle A1 centre (-15.5, 15.5) radius 1.5
  circle A2 centre (15.5, 15.5) radius 1.5
  circle A3 centre (-15.5, -15.5) radius 1.5
  line L0 (21.15, -18.85) -> (21.15, 18.85)
  line L1 (21.15, 18.85) -> (18.85, 21.15)
  line L2 (18.85, 21.15) -> (-18.85, 21.15)
  line L3 (-18.85, 21.15) -> (-21.15, 18.85)
  line L4 (-21.15, 18.85) -> (-21.15, -18.85)
  line L5 (-21.15, -18.85) -> (-18.85, -21.15)
  line L6 (-18.85, -21.15) -> (18.85, -21.15)
  line L7 (18.85, -21.15) -> (21.15, -18.85)
  circle A4 centre (0, 0) radius 11
  dimension "d17" = 22
  constraint coincident A4.centre origin
  measures "d17" diameter of A4
extrude "Extrude2" add sketch "Sketch2" along normal blind 2 contours A4
sketch "Sketch3" plane through (0, 0, 21.5) normal (0, 0, 1) x (-1, 0, 0)
  circle A0 centre (0, 0) radius 11
  circle A1 centre (0, 0) radius 2.5
  dimension "d20" = 5
  constraint coincident A0.centre A1.centre
  measures "d20" diameter of A1
extrude "Extrude3" add sketch "Sketch3" along normal blind 20 contours A1
sketch "Sketch4" plane through (0, 0, 41.5) normal (0, 0, 1) x (-1, 0, 0)
  circle A0 centre (0, 0) radius 2.5
  line L0 (1.2713, -2.1526) -> (-1.2713, -2.1526)
  arc A1 (-1.2713, -2.1526) -> (1.2713, -2.1526) centre (0, 0) ccw
  constraint coincident A0 L0.start
  constraint coincident A0 L0.end
  constraint horizontal L0
extrude "Extrude4" cut sketch "Sketch4" against normal blind 16 contours A0 L0 A1

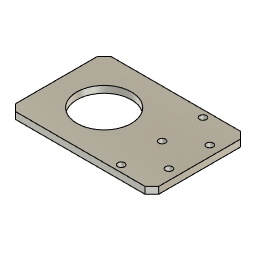
design "42减速输入固定"
Autodesk Fusion 360 part; units mm, degrees
sketch "草图1" plane through (0, 0, 0) normal (0, 0, 1) x (1, 0, 0)
  circle A0 centre (0, 0) radius 12
  line L0 (18, 21) -> (-18, 21)
  line L1 (-21, 18) -> (-21, -18)
  line L2 (-18, -21) -> (18, -21)
  line L3 (21, -18) -> (21, 18)
  line L4 (21, 21) -> (-21, -21) construction
  line L5 (-21, 21) -> (21, -21) construction
  circle A1 centre (15.5, -15.5) radius 1.75
  circle A2 centre (15.5, 15.5) radius 1.75
  circle A3 centre (-15.5, 15.5) radius 1.75
  circle A4 centre (-15.5, -15.5) radius 1.75
  line L6 (-18, 21) -> (-21, 18)
  line L7 (-21, -18) -> (-18, -21)
  line L8 (18, 21) -> (21, 18)
  line L9 (21, -18) -> (18, -21)
  line L10 (42, 18) -> (42, -18)
  line L11 (21, -18) -> (21, 18)
  line L12 (18, 21) -> (39, 21)
  line L13 (39, -21) -> (18, -21)
  circle A5 centre (25.5, 0) radius 1.5
  circle A6 centre (25.5, -18) radius 1.5
  circle A7 centre (37.5, -9) radius 1.5
  line L14 (79.2108, 0) -> (-40, 0) construction
  circle A8 centre (37.5, 9) radius 1.5
  circle A9 centre (25.5, 18) radius 1.5
  line L15 (39, 21) -> (42, 18)
  line L16 (42, -18) -> (39, -21)
  point P0 (42, 21)
  point P1 (42, -21)
  dimension "d1" = 24
  dimension "d2" = 42
  dimension "d3" = 42
  dimension "d4" = 15.5
  dimension "d5" = 3.5
  dimension "d7" = 360
  dimension "d8" = 3
  dimension "d9" = 3
  dimension "d10" = 3
  dimension "d11" = 3
  dimension "d12" = 3
  dimension "d13" = 3
  dimension "d14" = 3
  dimension "d15" = 3
  dimension "d17" = 21
  dimension "d20" = 3
  dimension "d21" = 3
  dimension "d22" = 3
  dimension "d24" = 18
  dimension "d25" = 9
  dimension "d26" = 4.5
  dimension "d27" = 4.5
  dimension "d28" = 16.5
  dimension "d32" = 3
  dimension "d33" = 3
  dimension "d34" = 3
  dimension "d35" = 3
  constraint coincident A0.centre origin
  constraint horizontal L0
  constraint perpendicular L0 L1
  constraint parallel L0 L2
  constraint parallel L1 L3
  constraint coincident L4 A0.centre
  constraint coincident L5 A0.centre
  constraint coincident L5 A1.centre
  constraint coincident L5.start L0
  constraint coincident L5.start L1
  constraint coincident L4.end L1
  constraint coincident L4.end L2
  constraint coincident L4.start L0
  constraint coincident L4.start L3
  constraint coincident L5.end L3
  constraint coincident L5.end L2
  constraint vertical L10
  constraint vertical L11
  constraint horizontal L12
  constraint horizontal L13
  constraint horizontal L14
  constraint coincident A0.centre L14
  constraint coincident A5.centre L14
  constraint symmetric A6 L14 A9
  constraint symmetric A7 L14 A8
  constraint coincident P0 L12
  constraint coincident P0 L10
  constraint coincident P1 L10
  constraint coincident P1 L13
  measures "d1" diameter of A0
  measures "d2" distance of L4.start L5.start
  measures "d3" distance of L4.start L5.end
  measures "d4" horizontal distance of A0.centre A1.centre
  measures "d5" diameter of A1
  measures "d8" distance of L5.start L0.end
  measures "d9" distance of L5.start L1.start
  measures "d10" distance of L4.end L1.end
  measures "d11" distance of L4.end L2.start
  measures "d12" distance of L4.start L0.start
  measures "d13" distance of L4.start L3.end
  measures "d14" distance of L5.end L3.start
  measures "d15" distance of L5.end L2.end
  measures "d17" distance of L10 L11
  measures "d20" diameter of A6
  measures "d21" diameter of A5
  measures "d22" diameter of A7
  measures "d24" distance of A6.centre L14
  measures "d25" distance of A7.centre L14
  measures "d26" distance of L11 A5.centre
  measures "d27" distance of L11 A6.centre
  measures "d28" distance of L3 A7.centre
  measures "d32" distance of P0 L12.end
  measures "d33" distance of P0 L10.start
  measures "d34" distance of P1 L10.end
  measures "d35" distance of P1 L13.start
extrude "拉伸1" add sketch "草图1" along normal blind 3 contours L0 L1 L2 L3 L6 L7 L8 L9 L11 | L3 L8 L9 L10 L11 L12 L13 L15 L16 | A1 | A2 | A3 | A4
extrude "拉伸2" add sketch "草图1" against normal blind 2 contours A1 | A2 | A3 | A4
chamfer "倒角1" distance 0.5 angle 45 4 edges at (13.8684, -14.8672, -2) (13.8684, 16.1328, -2) (-17.1316, 16.1328, -2) (-17.1316, -14.8672, -2)
equation "d9 = d8"
equation "d11 = d10"
equation "d13 = d12"
equation "d15 = d14"
equation "d33 = d32"
equation "d35 = d34"

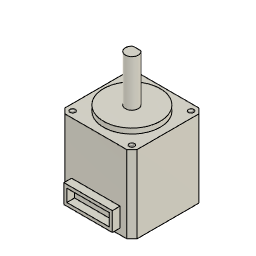
design "Motor_28*30"
Autodesk Fusion 360 part; units mm, degrees
sketch "草图1" plane through (0, 0, 0) normal (0, 0, 1) x (1, 0, 0)
  line L0 (12, 14) -> (-12, 14)
  line L1 (-14, 12) -> (-14, -12)
  line L2 (-12, -14) -> (12, -14)
  line L3 (14, -12) -> (14, 12)
  line L4 (14, 14) -> (-14, -14) construction
  line L5 (-14, 14) -> (14, -14) construction
  line L6 (12, 14) -> (14, 12)
  line L7 (14, -12) -> (12, -14)
  line L8 (-12, -14) -> (-14, -12)
  line L9 (-14, 12) -> (-12, 14)
  circle A0 centre (0, 0) radius 11
  circle A1 centre (0, 0) radius 2.5
  circle A2 centre (11.5, 11.5) radius 1.25
  circle A3 centre (-11.5, 11.5) radius 1.25
  circle A4 centre (-11.5, -11.5) radius 1.25
  circle A5 centre (11.5, -11.5) radius 1.25
  line L10 (-1.5, 2) -> (1.5, 2)
  dimension "d1" = 28
  dimension "d2" = 28
  dimension "d3" = 2
  dimension "d4" = 2
  dimension "d5" = 2
  dimension "d6" = 2
  dimension "d7" = 2
  dimension "d8" = 2
  dimension "d9" = 2
  dimension "d10" = 2
  dimension "d11" = 22
  dimension "d12" = 5
  dimension "d13" = 11.5
  dimension "d15" = 360
  dimension "d35" = 2.5
  dimension "d36" = 2
  constraint horizontal L0
  constraint perpendicular L0 L1
  constraint parallel L0 L2
  constraint parallel L1 L3
  constraint coincident L4 A0.centre
  constraint coincident L5 A0.centre
  constraint coincident A0.centre A1.centre
  constraint coincident L4.start L0
  constraint coincident L4.start L3
  constraint coincident L5.end L3
  constraint coincident L5.end L2
  constraint coincident L4.end L2
  constraint coincident L4.end L1
  constraint coincident L5.start L1
  constraint coincident L5.start L0
  constraint coincident L4 A2.centre
  constraint coincident A1 L10.start
  constraint coincident A1 L10.end
  constraint horizontal L10
  measures "d1" distance of L4.start L5.start
  measures "d2" distance of L4.start L5.end
  measures "d3" distance of L4.start L0.start
  measures "d4" distance of L4.start L3.end
  measures "d5" distance of L5.end L3.start
  measures "d6" distance of L5.end L2.end
  measures "d7" distance of L4.end L2.start
  measures "d8" distance of L4.end L1.end
  measures "d9" distance of L5.start L1.start
  measures "d10" distance of L5.start L0.end
  measures "d11" diameter of A0
  measures "d12" diameter of A1
  measures "d13" horizontal distance of A0.centre A2.centre
  measures "d35" diameter of A2
  measures "d36" distance of A0.centre L10
extrude "拉伸1" add sketch "草图1" against normal blind 30 contours L0 L1 L2 L3 L6 L7 L8 L9 | A0 | A1 L10 | A1 L10 | A2 | A3 | A4 | A5 makes body 1
extrude "拉伸2" add sketch "草图1" along normal blind 2 contours A0 | A1 L10 | A1 L10 bodies 1
extrude "拉伸3" add sketch "草图1" along normal blind 20 contours A1 L10 picked at (0.6865, -0.2754) bodies 1
split "分割1" by plane through (0, 0, 2) normal (0, 0, 1) bodies 1 makes body 2 at (-1.6884, 1.8437, 14)
copy_body "实体->零部件1" bodies 2 removing the originals makes body 3 in component "Component"
hole "孔1" at (11.5, 11.5, 0) at (11.5, -11.5, 0) at (-11.5, -11.5, 0) at (-11.5, 11.5, 0) direction (0, 0, -1) diameter 2.076 depth 10 tip angle 118 bodies 1
thread "螺纹1" "ISO Metric profile 2.5 M2.5x0.45 6H" major diameter 2.58 minor diameter 2.0755 pitch 0.45 angle 60 resizes the face on face at (-11.4483, 10.4633, -3.3333) on face at (11.5517, 10.4633, -3.3333) on face at (11.5517, -12.5367, -3.3333) on face at (-11.4483, -12.5367, -3.3333) on bodies 1
sketch "草图2" plane through (0, -14, 0) normal (0, -1, 0) x (1, 0, 0)
  line L0 (12, 0) -> (-12, 0)
  line L1 (-12, 0) -> (-12, -30)
  line L2 (-12, -30) -> (12, -30)
  line L3 (12, -30) -> (12, 0)
  line L4 (-9.4074, -27.6784) -> (9.4074, -27.6784)
  line L5 (9.4074, -27.6784) -> (9.4074, -20.3216)
  line L6 (9.4074, -20.3216) -> (-9.4074, -20.3216)
  line L7 (-9.4074, -20.3216) -> (-9.4074, -27.6784)
  line L8 (-9.4074, -27.6784) -> (9.4074, -20.3216) construction
  line L9 (9.4074, -27.6784) -> (-9.4074, -20.3216) construction
  line L10 (8.2453, -21.5991) -> (-8.2453, -21.5991)
  line L11 (-8.2453, -21.5991) -> (-8.2453, -26.4009)
  line L12 (-8.2453, -26.4009) -> (8.2453, -26.4009)
  line L13 (8.2453, -26.4009) -> (8.2453, -21.5991)
  line L14 (8.2453, -21.5991) -> (-8.2453, -26.4009) construction
  line L15 (-8.2453, -21.5991) -> (8.2453, -26.4009) construction
  line L16 (0, 0) -> (0, -24) construction
  point P0 (0, -24)
  point P1 (0, -24)
  constraint horizontal L4
  constraint perpendicular L4 L5
  constraint parallel L4 L6
  constraint parallel L5 L7
  constraint coincident L8 P1
  constraint coincident L9 P1
  constraint horizontal L10
  constraint perpendicular L10 L11
  constraint parallel L10 L12
  constraint parallel L11 L13
  constraint coincident L14 P1
  constraint coincident L15 P1
  constraint coincident P1 P0
  constraint coincident L16.start origin
  constraint vertical L16
extrude "拉伸4" add sketch "草图2" along normal blind 3 contours L4 L5 L6 L7 bodies 1
component "Component" placed x (1, 0, 0) y (0, 1, 0) z (0, 0, 1) at (0, 0, 0)

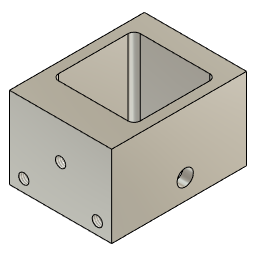
design "铝型连28"
Autodesk Fusion 360 part; units mm, degrees